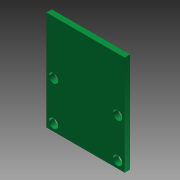
# Autodesk Inventor part: Encoder
Saved by Autodesk Inventor 2014 SP1 (Build 180222100, 222)
## iProperties
Created: 2012-02-19
Part Number: Encoder
Material: Generic
Document SubType Name: Modeling
Designer: Moses
Mass: 0.904144 g
Surface Area: 14.0253 cm^2
Volume: 0.904144 cm^3
Density: 1 g/cm^3
Appearance: Smooth - Dark Forest Green
Author: Moses
Autodesk Inventor part; units mm, degrees
ref_plane "YZ Plane" through (0, 0, 0) normal (1, 0, 0) x (0, 1, 0)
ref_plane "XZ Plane" through (0, 0, 0) normal (0, 1, 0) x (-1, 0, 0)
ref_plane "XY Plane" through (0, 0, 0) normal (0, 0, 1) x (1, 0, 0)
sketch "Sketch1" plane through (0, 0, 0) normal (0, 0, 1) x (1, 0, 0)
  line L0 (0, 0) -> (0, 28)
  line L1 (0, 28) -> (22, 28)
  line L2 (22, 28) -> (22, 0)
  line L3 (22, 0) -> (0, 0)
  circle A0 centre (2, 13) radius 1.3
  circle A1 centre (20, 13) radius 1.3
  circle A2 centre (2, 2) radius 1.3
  circle A3 centre (20, 2) radius 1.3
  line L4 (11, 28) -> (11, 0) construction
  line L5 (2, 13) -> (20, 13) construction
  line L6 (2, 2) -> (20, 2) construction
  line L7 (9, 9) -> (13, 9)
  line L8 (13, 9) -> (13, 6)
  line L9 (13, 6) -> (9, 6)
  line L10 (9, 6) -> (9, 9)
  line L11 (2, 13) -> (2, 2)
  line L12 (9, 7.5) -> (13, 7.5) construction
  line L13 (11, 13) -> (11, 2) construction
  point P0 (11, 9)
  point P1 (11, 7.5)
  dimension "d0" = 28
  dimension "d1" = 22
  dimension "d2" = 2.6
  dimension "d5" = 18
  dimension "d8" = 11
  dimension "d11" = 2
  dimension "d14" = 4
  dimension "d15" = 3
  constraints: 28 end point, 9 midpoint, 6 perpendicular, 4 centre point, 3 parallel, 2 horizontal, 2 point on line, 2 vertical, 1 collinear, 6 other
  measures "d0" distance of L0.start L0.end
  measures "d1" distance of L0.end L1.end
  measures "d2" diameter of A0
  measures "d5" distance of L5.start L5.end
  measures "d8" distance of L5.start L6.start
  measures "d11" distance between parallel lines of L3 L6
  measures "d14" distance of L7.start L7.end
  measures "d15" distance of L7.end L8.end
extrude "Extrusion1" add sketch "Sketch1" along normal blind 1.5 contours L0 L1 L2 L3 | L7 L8 L9 L10
extrude "Extrusion2" add sketch "Sketch1" against normal blind 1 contours L7 L8 L9 L10
body "Solid1"
